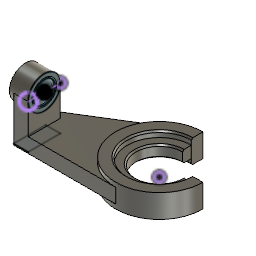
hw2 (Autodesk Fusion 360 design; units mm, degrees)
part number: 2026-08-05-13-20-17-199
Autodesk Fusion 360 part; units mm, degrees
sketch "스케치1" plane through (0, 0, 0) normal (0, 0, 1) x (1, 0, 0)
  circle A0 centre (0, 0) radius 16
  circle A1 centre (0, 0) radius 22
  circle A2 centre (0, 0) radius 30
  line L0 (0, 0) -> (0, -30) construction
  line L1 (-15.7735, 25.5185) -> (-70, -8)
  line L2 (-70, -8) -> (-70, -30)
  line L3 (-70, -30) -> (0, -30)
  dimension "d1" = 32
  dimension "d2" = 44
  dimension "d3" = 60
  dimension "d18" = 70
  dimension "d19" = 22
  constraint coincident A0.centre A1.centre
  constraint concentric A0 A1
  constraint tangent A2 L1
  constraint coincident A2 L1.start
  constraint vertical L2
  constraint horizontal L3
  constraint tangent A2 L3
  constraint coincident A2 L0.end
  measures "d1" diameter of A0
  measures "d2" diameter of A1
  measures "d3" diameter of A2
  measures "d18" horizontal distance of A0.centre L1.end
  measures "d19" distance of L1.end L2.end
extrude "돌출1" add sketch "스케치1" along normal blind 8 contours A2 makes body 1
extrude "돌출2" add sketch "스케치1" along normal blind 4 separate body contours A1 makes body 2
chamfer "챔퍼1" distance 1 angle 45 1 edges at (-20.5112, 7.9555, 8) on bodies 1
chamfer "챔퍼2" distance 1 angle 45 1 edges at (-14.9172, 5.7858, 4) measured on face at (19.8585, -1.8879, 4) on bodies 2
sketch "스케치2" plane through (0, 0, 0) normal (0, 0, 1) x (1, 0, 0)
  line L0 (0, 0) -> (30, 0)
  line L1 (30, 0) -> (30, 30)
  line L2 (30, 30) -> (0, 30)
  line L3 (0, 30) -> (0, 0)
  dimension "d11" = 30
  dimension "d12" = 30
  constraint horizontal L0
  constraint vertical L1
  constraint horizontal L2
  constraint vertical L3
  constraint coincident L0.start L3.end
  measures "d11" distance of L0.start L0.end
  measures "d12" distance of L0.start L2.end
mirror "미러2" about plane through (0, 0, 0) normal (0, 0, 1) of bodies 1 2 merged
extrude "돌출11" cut sketch "스케치2" along normal mid plane 16 bodies 1 2
extrude "돌출12" add sketch "스케치1" along normal mid plane 10 contours A2 L1 L2 L3 bodies 1
ref_plane "작업 평면3" through (0, 0, -4) normal (0, 0, -1) x (1, 0, 0)
sketch "스케치19" plane through (0, 0, -4) normal (0, 0, -1) x (-1, 0, 0)
  line L0 (70, -30) -> (60, -30)
  line L1 (60, -30) -> (60, -8)
  line L2 (60, -8) -> (70, -8)
  line L3 (70, -8) -> (70, -30)
  dimension "d75" = 10
  dimension "d76" = 22
  dimension "d77" = 70
  dimension "d78" = 30
  constraint horizontal L0
  constraint vertical L1
  constraint horizontal L2
  constraint vertical L3
  measures "d75" distance of L0.start L0.end
  measures "d76" distance of L0.start L2.end
  measures "d77" horizontal distance of origin L2.end
  measures "d78" distance of origin L0
extrude "돌출15" add sketch "스케치19" against normal blind 30 bodies 1
ref_plane "작업 평면4" through (-60, -19, 15.5) normal (1, 0, 0) x (0, 1, 0)
sketch "스케치20" plane through (-60, 0, 0) normal (1, 0, 0) x (0, 1, 0)
  circle A0 centre (-19, 26) radius 11
  circle A1 centre (-19, 26) radius 7.5
  line L0 (-30, 26) -> (-8, 26)
  dimension "d83" = 22
  dimension "d84" = 15
  constraint concentric A0 A1
  constraint coincident A0.centre L0
  constraint coincident A0 L0.end
  measures "d83" diameter of A0
  measures "d84" diameter of A1
extrude "돌출16" add sketch "스케치20" against normal blind 13 contours A0 A1 L0 picked at (-26.783, 31.9678) bodies 1
extrude "돌출17" add sketch "스케치20" against normal blind 13 contours A0 A1 L0 picked at (-9.2355, 25.0809) bodies 1
extrude "돌출18" cut sketch "스케치20" against normal blind 10 contours A1 L0 picked at (-18.4437, 23.5627) bodies 1
chamfer "챔퍼3" distance 1 angle 45 1 edges at (-60, -25.9925, 28.7121) on bodies 1
chamfer "챔퍼4" distance 1 angle 45 1 edges at (-73, -25.9925, 23.2879) on bodies 1
